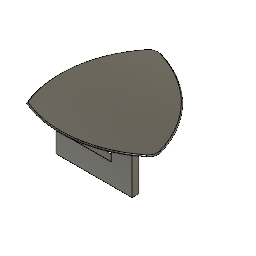
coffee table (Autodesk Fusion 360 design; units mm, degrees)
Autodesk Fusion 360 part; units mm, degrees
sketch "Blueprint" plane through (0, 0, 0) normal (0, 0, 1) x (1, 0, 0)
  line L0 (0, 0) -> (110, 0)
  line L1 (0, 0) -> (0, 110)
  line L2 (0, 110) -> (10, 110)
  line L3 (10, 110) -> (10, 0)
  line L4 (110, 0) -> (110, 10)
  line L5 (110, 10) -> (10, 10)
  line L6 (5, 110) -> (5, 140) construction
  line L7 (110, 5) -> (140, 5) construction
  line L8 (0, 0) -> (-21.2132, -21.2132) construction
  line L9 (0, 0) -> (30, 0) construction
  circle A0 centre (5, 125) radius 15 construction
  circle A1 centre (-10.6066, -10.6066) radius 15 construction
  circle A2 centre (125, 5) radius 15 construction
  arc A3 (-1.4696, 132.3743) -> (-21.2132, -21.2132) centre (116.0829, 39.2002) ccw construction
  arc A4 (-21.2132, -21.2132) -> (132.3743, -1.4696) centre (39.2002, 116.0829) ccw construction
  arc A5 (137.4337, 14.5645) -> (14.5645, 137.4337) centre (-37.5, -37.5) ccw construction
  arc A6 (14.5645, 137.4337) -> (-1.4696, 132.3743) centre (10.2856, 123.0569) ccw construction
  arc A7 (132.3743, -1.4696) -> (137.4337, 14.5645) centre (123.0569, 10.2856) ccw construction
  dimension "d1" = 135
  dimension "d2" = 30
  dimension "d3" = 150
  dimension "d4" = 182.5171
  dimension "d5" = 15
  dimension "d6" = 15
  constraint coincident L0.start L1.start
  constraint horizontal L0
  constraint perpendicular L0 L1
  constraint perpendicular L1 L2
  constraint coincident L0 L3.end
  constraint perpendicular L2 L3
  constraint perpendicular L0 L4
  constraint coincident L3 L5.end
  constraint perpendicular L3 L5
  constraint midpoint L2 L6.start
  constraint perpendicular L2 L6
  constraint midpoint L4 L7.start
  constraint perpendicular L4 L7
  constraint horizontal L9
  constraint midpoint L6 A0.centre
  constraint midpoint L8 A1.centre
  constraint coincident L8.end A1
  constraint midpoint L7 A2.centre
  constraint coincident L7.end A2
  constraint symmetric A3.end L8 A4.start
  constraint symmetric L8 A3 A4
  constraint coincident L6.end A5
  constraint tangent A5 A6
  constraint tangent A3 A6
  constraint tangent A4 A7
  constraint tangent A5 A7
  measures "d1" angle of L8 L9
  measures "d2" distance of L0.start L8.end
  measures "d3" radius of A3
  measures "d4" radius of A5
  measures "d5" radius of A6
  measures "d6" radius of A7
extrude "Extrude1" add sketch "Blueprint" along normal blind 60 makes body 1
sketch "Side 1" plane through (0, 0, 0) normal (-1, 0, 0) x (0, -1, 0)
  line L0 (-110, 0) -> (0, 0)
  line L1 (0, 0) -> (0, 60)
  line L2 (0, 60) -> (-110, 60)
  line L3 (-110, 60) -> (-110, 0)
  line L4 (0, 0) -> (-10, 0) construction
  line L5 (0, 60) -> (-10, 60) construction
  line L6 (-10, 60) -> (-10, 0) construction
  line L7 (-110, 0) -> (-80, 0) construction
  line L8 (-110, 30) -> (0, 30) construction
  line L9 (-80, 0) -> (-10, 0)
  line L10 (-10, 0) -> (-10, 30)
  line L11 (-10, 30) -> (-80, 30)
  line L12 (-80, 30) -> (-80, 0)
  constraint coincident L0.end L1.start
  constraint coincident L0 L4.end
  constraint perpendicular L1 L4
  constraint coincident L1.end L2.start
  constraint coincident L2 L5.end
  constraint perpendicular L1 L5
  constraint perpendicular L0 L6
  constraint coincident L0.start L3.end
  constraint coincident L0 L7.end
  constraint midpoint L3 L8.start
  constraint midpoint L1 L8.end
  constraint horizontal L9
  constraint vertical L10
  constraint horizontal L11
  constraint vertical L12
  constraint midpoint L6 L10.end
extrude "Extrude2" cut sketch "Side 1" against normal blind 20 contours L0 L9 L10 L11 L12 bodies 1
ref_plane "WorkPlane1" through (5, 45, 30) normal (0, 0, -1) x (0, 1, 0)
sketch "Side 2" plane through (0, 10, 0) normal (0, 1, 0) x (-1, 0, 0)
  line L0 (-10, 30) -> (-10, 60)
  line L1 (-10, 60) -> (-110, 60)
  line L2 (-110, 60) -> (-110, 0)
  line L3 (-110, 0) -> (0, 0)
  line L4 (0, 0) -> (0, 30)
  line L5 (0, 30) -> (-10, 30)
  line L6 (-110, 60) -> (-80, 60) construction
  line L7 (-80, 0) -> (-80, 60) construction
  line L8 (-10, 30) -> (-80, 30)
  line L9 (-80, 60) -> (-80, 30)
  constraint coincident L1.end L2.start
  constraint coincident L1 L6.end
  constraint perpendicular L2 L6
  constraint coincident L3 L7.start
  constraint perpendicular L1 L7
  constraint coincident L0.start L5.end
  constraint midpoint L7 L8.end
extrude "Extrude3" cut sketch "Side 2" against normal blind 40 contours L0 L1 L8 L9 bodies 1
sketch "Sketch5" plane through (0, 0, 0) normal (-1, 0, 0) x (0, -1, 0)
sketch "Cirlcles" plane through (0, 0, 60) normal (0, 0, 1) x (-1, 0, 0)
  line L0 (-80, -10) -> (-80, 0)
  line L1 (-80, 0) -> (-110, 0)
  line L2 (-110, 0) -> (-110, -10)
  line L3 (-110, -10) -> (-80, -10)
  circle A0 centre (-100, -5) radius 4
  circle A1 centre (-5, -5) radius 4
  line L4 (-110, -5) -> (-100, -5) construction
  line L5 (-5, -110) -> (-5, -100) construction
  circle A2 centre (-5, -100) radius 4
  dimension "d14" = 8
  constraint midpoint L2 L4.start
  constraint coincident A0.centre L4.end
  constraint vertical L5
  constraint coincident L5.end A2.centre
  measures "d14" diameter of A2
extrude "Extrude4" add sketch "Cirlcles" along normal blind 2 contours A0 | A1 | A2 bodies 1
sketch "Separating points " plane through (5, 45, 30) normal (0, 0, -1) x (1, 0, 0)
  point P0 (-5, 35)
  point P1 (-5, 45)
  point P2 (5, 45)
  point P3 (5, 35)
sketch "Sketch8" plane through (0, 0, 62) normal (0, 0, 1) x (-1, 0, 0)
  circle A0 centre (-5, -5) radius 4
  arc A1 (1.4696, -132.3743) -> (21.2132, 21.2132) centre (-116.0829, -39.2002) ccw
  arc A2 (21.2132, 21.2132) -> (-132.3743, 1.4696) centre (-39.2002, -116.0829) ccw
  arc A3 (-137.4337, -14.5645) -> (-14.5645, -137.4337) centre (37.5, 37.5) ccw
  arc A4 (-14.5645, -137.4337) -> (1.4696, -132.3743) centre (-10.2856, -123.0569) ccw
  arc A5 (-132.3743, 1.4696) -> (-137.4337, -14.5645) centre (-123.0569, -10.2856) ccw
surface "SurfacePatch1" add patch path "Sketch8" along A3 A4 A1 A2 A5 separate body makes body 2
thicken "Thicken1" add thickness 2.5 1 faces at (28.7405, 34.8334, 62) separate body on bodies 2 makes body 3
fillet "Fillet1" radius 1.4 5 edges at (58.3253, -32.6929, 64.5) (137.3617, 5.772, 64.5) (91.5591, 91.5591, 64.5) (5.772, 137.3617, 64.5) (-32.6929, 58.3253, 64.5) on bodies 3
fillet "Fillet2" radius 2 5 edges at (58.3253, -32.6929, 62) (137.3617, 5.772, 62) (91.5591, 91.5591, 62) (5.772, 137.3617, 62) (-32.6929, 58.3253, 62) on bodies 3
hidden bodies 2
